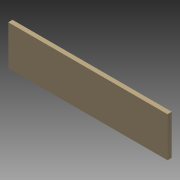
# Autodesk Inventor part: back crossboard
Saved by Autodesk Inventor 2012 (Build 160160000, 160)
## iProperties
Created: 2013-05-09
Part Number: back crossboard
Material: Default
Document SubType Name: Modeling
Designer: Fabian
Density: 1 g/cm^3
Author: Fabian
Autodesk Inventor part; units mm, degrees
ref_plane "YZ Plane" through (0, 0, 0) normal (1, 0, 0) x (0, 1, 0)
ref_plane "XZ Plane" through (0, 0, 0) normal (0, 1, 0) x (-1, 0, 0)
ref_plane "XY Plane" through (0, 0, 0) normal (0, 0, 1) x (1, 0, 0)
sketch "Sketch1" plane through (0, 0, 0) normal (0, 0, 1) x (1, 0, 0)
  line L0 (-25.2448, 97.4741) -> (685.9552, 97.4741)
  line L1 (685.9552, 97.4741) -> (685.9552, -80.3259)
  line L2 (685.9552, -80.3259) -> (-25.2448, -80.3259)
  line L3 (-25.2448, -80.3259) -> (-25.2448, 97.4741)
  point P0 (0, 0)
  dimension "d0" = 177.8
  dimension "d1" = 711.2
  constraints: 8 end point, 2 parallel, 1 horizontal, 1 perpendicular
  measures "d0" distance of L2.end L0.start
  measures "d1" distance of L0.start L0.end
extrude "Extrusion1" add sketch "Sketch1" along normal blind 19.05
body "Solid1"
